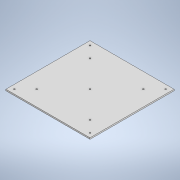
# Autodesk Inventor part: Plate
Saved by Autodesk Inventor 2020.3 (Build 243373010, 373A)
## iProperties
Created: 2020-10-30
Part Number: Plate
Material: Generic
Document SubType Name: Modeling
Designer: Naude Conradie
Density: 1 g/cm^3
Appearance: Default
Author: Naude Conradie
Autodesk Inventor part; units mm, degrees
ref_plane "YZ Plane" through (0, 0, 0) normal (1, 0, 0) x (0, 1, 0)
ref_plane "XZ Plane" through (0, 0, 0) normal (0, 1, 0) x (-1, 0, 0)
ref_plane "XY Plane" through (0, 0, 0) normal (0, 0, 1) x (1, 0, 0)
sketch "Sketch1" plane through (0, 0, 0) normal (0, 1, 0) x (-1, 0, 0)
  line L0 (0, 0) -> (300, 0)
  line L1 (300, 0) -> (300, -300)
  line L2 (300, -300) -> (0, -300)
  line L3 (0, -300) -> (0, 0)
  dimension "d0" = 300
  dimension "d1" = 300
  constraints: 8 end point, 2 parallel, 1 horizontal, 1 perpendicular
  measures "d0" distance of L1.end L2.end
  measures "d1" distance of L0.end L1.end
extrude "Extrusion1" add sketch "Sketch1" along normal blind 5
sketch "Sketch2" plane through (0, 5, 0) normal (0, 1, 0) x (1, 0, 0)
  line L0 (-300, 0) -> (0, 0) projected
  line L1 (0, 0) -> (0, 300) projected
  point P0 (-15, 15)
  point P1 (-15, 285)
  point P2 (-285, 15)
  point P3 (-285, 285)
  dimension "d4" = 15
  dimension "d5" = 15
  dimension "d8" = 270
  dimension "d11" = 270
  constraints: 1 horizontal, 1 vertical, 3 other
  measures "d4" horizontal distance of L0.end point (-15, 15)
  measures "d5" horizontal distance of L0.end point (-15, 15)
  measures "d8" distance of point (-15, 15) point (-15, 285)
  measures "d11" distance of point (-15, 15) point (-285, 15)
hole "Hole1" at (-15, 5, -15) at (-15, 5, -285) at (-285, 5, -15) at (-285, 5, -285) direction (0, -1, 0) diameter 5 end through all
sketch "Sketch3" plane through (0, 5, 0) normal (0, 1, 0) x (1, 0, 0)
  line L0 (-300, 300) -> (-300, 0) projected
  line L1 (0, 300) -> (-300, 300) projected
  point P0 (0, 0)
  point P1 (-150, 150)
  point P2 (-245, 245)
  point P3 (-245, 55)
  point P4 (-55, 245)
  point P5 (-55, 55)
  dimension "d21" = 150
  dimension "d22" = 150
  dimension "d23" = 55
  dimension "d26" = 190
  dimension "d29" = 190
  dimension "d32" = 55
  constraints: 1 horizontal, 1 vertical, 3 other
  measures "d21" horizontal distance of point (0, 0) point (-150, 150)
  measures "d22" horizontal distance of point (0, 0) point (-150, 150)
  measures "d23" distance from line of L0 point (-245, 245)
  measures "d26" distance of point (-245, 245) point (-245, 55)
  measures "d29" distance of point (-245, 245) point (-55, 245)
  measures "d32" distance from line of L1 point (-245, 245)
hole "Hole2" at (-150, 5, -150) at (-245, 5, -245) at (-245, 5, -55) at (-55, 5, -245) at (-55, 5, -55) direction (0, -1, 0) diameter 5 end through all
body "Solid1"
